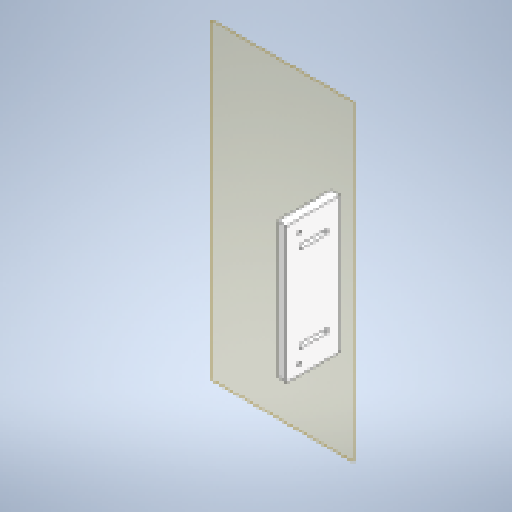
# Autodesk Inventor part: 60
Saved by Autodesk Inventor 2024.3 (Build 283343000, 343)
## iProperties
Created: 2024-09-08
Part Number: 60
Material: 아크릴, 선명
Document SubType Name: Modeling
Designer: 구지현
Density: 1.19 g/cm^3
Appearance: 흰색
Author: 구지현
Autodesk Inventor part; units mm, degrees
ref_plane "YZ Plane" through (0, 0, 0) normal (1, 0, 0) x (0, 1, 0)
ref_plane "XZ Plane" through (0, 0, 0) normal (0, 1, 0) x (-1, 0, 0)
ref_plane "XY Plane" through (0, 0, 0) normal (0, 0, 1) x (1, 0, 0)
ref_plane "작업 평면1" through (0, 0, 0) normal (0, 0, 1) x (1, 0, 0)
sketch "스케치1" plane through (0, 0, 0) normal (0, 0, 1) x (1, 0, 0)
  line L0 (42.4906, -94.9526) -> (42.4906, 93.0474) projected
  line L1 (42.4906, 93.0474) -> (-42.5094, 93.0474) projected
  line L2 (-42.5094, 93.0474) -> (-42.5094, -94.9526) projected
  line L3 (-42.5094, -94.9526) -> (42.4906, -94.9526) projected
  line L4 (0, 0) -> (0, 35)
  line L5 (0, 0) -> (25, 0)
  line L6 (0, 0) -> (0, -35)
  line L7 (0, 0) -> (-25, 0)
  line L8 (25, 35) -> (-25, 35)
  line L9 (-25, 35) -> (-25, -35)
  line L10 (-25, -35) -> (25, -35)
  line L11 (25, -35) -> (25, 35)
  line L12 (35, 45) -> (-35, 45)
  line L13 (-35, 45) -> (-35, -45)
  line L14 (-35, -45) -> (35, -45)
  line L15 (35, -45) -> (35, 45)
  line L16 (35, 45) -> (38, 45)
  line L17 (38, 45) -> (32, 45)
  line L18 (32, 45) -> (32, -45)
  line L19 (32, -45) -> (38, -45)
  line L20 (38, -45) -> (38, 45)
  line L21 (-35, 45) -> (-38, 45)
  line L22 (-38, 45) -> (-38, 42)
  line L23 (-38, 42) -> (-35, 42)
  line L24 (-35, 42) -> (-35, 45)
  line L25 (-38, 45) -> (-32, 45)
  line L26 (-32, 45) -> (-32, -45)
  line L27 (-32, -45) -> (-38, -45)
  line L28 (-38, -45) -> (-38, 45)
  circle A0 centre (7, -59) radius 1.25 projected
  circle A1 centre (-1, 59) radius 1.25 projected
  circle A2 centre (-1, -59) radius 1.25 projected
  circle A3 centre (7, 59) radius 1.25 projected
  dimension "d0" = 35
  dimension "d1" = 25
  dimension "d2" = 35
  dimension "d3" = 25
  dimension "d4" = 10
  dimension "d5" = 3
  dimension "d6" = 6
  dimension "d7" = 3
  dimension "d8" = 3
  dimension "d9" = 6
  constraints: 50 end point, 10 parallel, 6 horizontal, 5 perpendicular, 3 point on line, 2 vertical, 3 other
  measures "d0" distance of L4.start L4.end
  measures "d1" distance of L4.start L5.end
  measures "d2" distance of L4.start L6.end
  measures "d3" distance of L4.start L7.end
  measures "d4" distance between parallel lines of L11 L15
  measures "d5" distance of L12.start L16.end
  measures "d6" distance of L19.end L18.end
  measures "d7" distance of L23.end L22.end
  measures "d8" distance of L22.end L21.end
  measures "d9" distance of L26.end L27.end
extrude "돌출1" add sketch "스케치1" along normal blind 35 contours L15 L14 L18 L12 | L16 L20 L19 L15
sketch "스케치2" plane through (38, -45, 0) normal (1, 0, 0) x (0, 0, -1)
  circle A0 centre (-27, 82) radius 1.25 projected
  line L0 (-22, 77) -> (-32, 77) projected
  line L1 (-32, 77) -> (-32, 87) projected
  line L2 (-32, 87) -> (-22, 87) projected
  line L3 (-22, 87) -> (-22, 77) projected
  circle A1 centre (-27, 6.5) radius 1.25 projected
  line L4 (-32, 3) -> (-32, 10) projected
  line L5 (-22, 10) -> (-32, 10) projected
  line L6 (-22, 3) -> (-22, 10) projected
  line L7 (-32, 3) -> (-22, 3) projected
  point P0 (0, 45)
extrude "돌출2" cut sketch "스케치2" against normal blind 35 contours A0 | A1
sketch "스케치3" plane through (38, -45, 0) normal (1, 0, 0) x (0, 0, -1)
  circle A0 centre (-27, 82) radius 1.25 projected
  circle A1 centre (-27, 6.5) radius 1.25 projected
  line L0 (0, 0) -> (0, 90) projected
  line L1 (0, 90) -> (-35, 90) projected
  line L2 (-35, 0) -> (-35, 90) projected
  line L3 (0, 0) -> (-35, 0) projected
  line L4 (0, 0) -> (-35, 0) projected
  line L5 (-35, 0) -> (-35, 90) projected
  line L6 (0, 0) -> (0, 90) projected
  line L7 (-27, 15) -> (-8, 15)
  line L8 (-8, 15) -> (-8, 18)
  line L9 (-8, 18) -> (-27, 18)
  line L10 (-27, 18) -> (-27, 15)
  line L11 (0, 90) -> (-35, 90) projected
  line L12 (-27, 75) -> (-8, 75)
  line L13 (-8, 75) -> (-8, 72)
  line L14 (-8, 72) -> (-27, 72)
  line L15 (-27, 72) -> (-27, 75)
  point P0 (0, 45)
  point P1 (-18.9095, 15)
  point P2 (-17.5, 0)
  point P3 (-8, 18.9545)
  point P4 (-18.9095, 75)
  point P5 (-17.5, 90)
  point P6 (-27, 64.4269)
  dimension "d14" = 15
  dimension "d15" = 8
  dimension "d16" = 8
  dimension "d17" = 3
  dimension "d18" = 15
  dimension "d19" = 8
  dimension "d20" = 3
  constraints: 16 end point, 4 parallel, 2 horizontal, 2 midpoint, 2 perpendicular
  measures "d14" vertical distance of point (-17.5, 0) point (-18.91, 15)
  measures "d15" distance from line of L7.start L5
  measures "d16" distance from line of L6 point (-8, 18.954)
  measures "d17" distance of L8.end L7.end
  measures "d18" vertical distance of point (-17.5, 90) point (-18.91, 75)
  measures "d19" distance from line of point (-27, 64.427) L5
  measures "d20" distance of L12.end L13.end
extrude "돌출3" cut sketch "스케치3" against normal blind 35 contours L10 L9 L8 L7 | L12 L13 L14 L15
